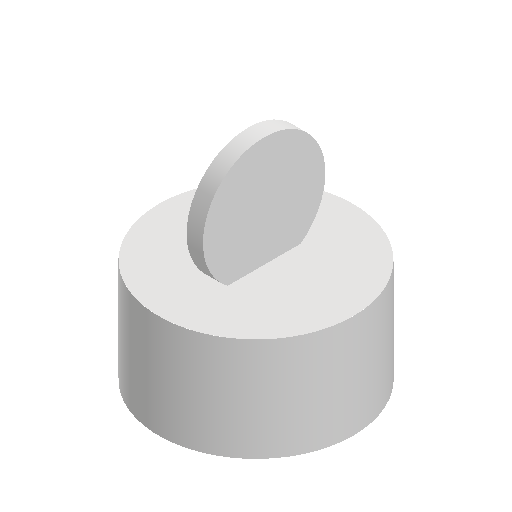
# Autodesk Inventor part: 萬向頭
Saved by Autodesk Inventor 2025.2 (Build 292293000, 293)
## iProperties
Created: 2025-07-21
Part Number: 萬向頭
Material: 一般
Document SubType Name: Modeling
Designer: jna1j
Density: 1 g/cm^3
Appearance: 預設
Author: jna1j
Autodesk Inventor part; units mm, degrees
ref_plane "YZ Plane" through (0, 0, 0) normal (1, 0, 0) x (0, 1, 0)
ref_plane "XZ Plane" through (0, 0, 0) normal (0, 1, 0) x (-1, 0, 0)
ref_plane "XY Plane" through (0, 0, 0) normal (0, 0, 1) x (1, 0, 0)
sketch "草圖1" plane through (0, 0, 0) normal (0, 1, 0) x (-1, 0, 0)
  circle A0 centre (0, 0) radius 5
  dimension "d0" = 10
  constraints: 1 centre point, 1 coincident
  measures "d0" diameter of A0
extrude "擠出1" add sketch "草圖1" along normal blind 5.32
sketch "草圖2" plane through (0, 0, 0) normal (1, 0, 0) x (0, 1, 0)
  circle A0 centre (7.85, 0) radius 3.15
  line L0 (0, 0) -> (11, 0)
  dimension "d3" = 6.3
  dimension "d4" = 11
  constraints: 2 end point, 2 horizontal alignment, 1 horizontal, 2 other
  measures "d4" distance of L0.start L0.end
extrude "擠出2" add sketch "草圖2" along normal mid plane 0.84
